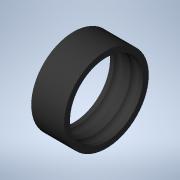
# Autodesk Inventor part: hpc_Q2307-ACC_1
Saved by Autodesk Inventor 2021 (Build 250183000, 183)
## iProperties
Created: 2026-05-26
Part Number: hpc_Q2307-ACC_1
Material: Generic
Catalog Web Link: www.3dfindit.com
Description: Q1Q2-1-Roulement à rotule sur billes - acier
Vendor: HPC
Document SubType Name: Modeling
Designer: psAdmin
Manufacturer: HPC
Mass: 37.6895 g
Surface Area: 173.998 cm^2
Volume: 37.6895 cm^3
Density: 1 g/cm^3
Appearance: PSOLRGB-176-176-176
Category: PARTsolutions
Company: HPC
Title: HPC - Q2307-ACC
Author: Cadenas PARTsolutions
Comments: Roulement à rotule sur billes - acier
PSOL_IDENT_0: {$CADENAS_DATA/23d-libs/hpc/v3/rotary/radial/steel/q1q2/q1q2_1.prj},171 {VTYP=3D},{NB=hpc_Q2307-ACC_
PSOL_IDENT_1: 1},{LINA=HPC - Q2307-ACC},{NN=Q1Q2-1},{DATE=26.05.2021 13:15:38},{GEOMDATE=24.09.2019 07:57:00},{VER
PSOL_IDENT_2: SION=},{LINEID=220},{WBVAR=},{WBNUMERIC=}  {NB=hpc_Q2307-ACC_1},{LINA=HPC - Q2307-ACC},{KT=DUMMY},{R
PSOL_IDENT_3: EF=Q2307-ACC},{D=35},{D1=80},{B=31},{CD=38.91},{CS=10.98},{VLG=9180},{VLH=10800},{MAS=0.680},{INFO=I
PSOL_IDENT_4: NFO}
NB: hpc_Q2307-ACC_1
NN: Q1Q2-1
NT: Roulement à rotule sur billes - acier
NBSYN: hpc_$REF._1
LINA: HPC - Q2307-ACC
CATALOG: HPC
REF: Q2307-ACC
D: 35
D1: 80
B: 31
CD: 38.91
CS: 10.98
VLG: 9180
VLH: 10800
MAS: 0.68
INFO: INFO
SUPPLIER: HPC
ARTICLENO: hpc_Q2307-ACC_1
BOMINFO: HPC - Q2307-ACC
CREATOR: CADENAS GmbH
Autodesk Inventor part; units mm, degrees
sketch "Sketch_1" plane through (0, 0, 0) normal (0, 0, 1) x (1, 0, 0)
  line L0 (50, 0) -> (-50, 0)
  line L1 (0, 34.3864) -> (3.2698, 34.3864)
  arc A0 (3.2698, 34.3864) -> (4.1774, 34.6401) centre (3.2698, 36.1364) ccw
  arc A1 (11.3226, 34.6401) -> (4.1774, 34.6401) centre (7.75, 28.75) ccw
  arc A2 (11.3226, 34.6401) -> (12.2302, 34.3864) centre (12.2302, 36.1364) ccw
  line L2 (12.2302, 34.3864) -> (18.7698, 34.3864)
  arc A3 (18.7698, 34.3864) -> (19.6774, 34.6401) centre (18.7698, 36.1364) ccw
  arc A4 (26.8226, 34.6401) -> (19.6774, 34.6401) centre (23.25, 28.75) ccw
  arc A5 (26.8226, 34.6401) -> (27.7302, 34.3864) centre (27.7302, 36.1364) ccw
  line L3 (27.7302, 34.3864) -> (31, 34.3864)
  line L4 (31, 34.3864) -> (31, 40)
  line L5 (31, 40) -> (0, 40)
  line L6 (0, 40) -> (0, 34.3864)
  constraints: 14 end point, 12 point on circle, 6 centre point
revolve "Revolution1" add sketch "Sketch_1" angle 360 about axis through (50, 0, 0) along (1, 0, 0)
ref_plane "IP_1_XY" through (0, 0, 0) normal (1, 0, 0) x (0, 0, -1)
ref_plane "IP_1_YZ" through (0, 0, 0) normal (0, 0, -1) x (0, 1, 0)
ref_plane "IP_1_ZX" through (0, 0, 0) normal (0, 1, 0) x (1, 0, 0)
ref_plane "IP_2_XY" through (15.5, 0, 0) normal (1, 0, 0) x (0, 0, -1)
ref_plane "IP_2_YZ" through (15.5, 0, 0) normal (0, 0, -1) x (0, 1, 0)
ref_plane "IP_2_ZX" through (15.5, 0, 0) normal (0, 1, 0) x (1, 0, 0)
body "Solid1"
